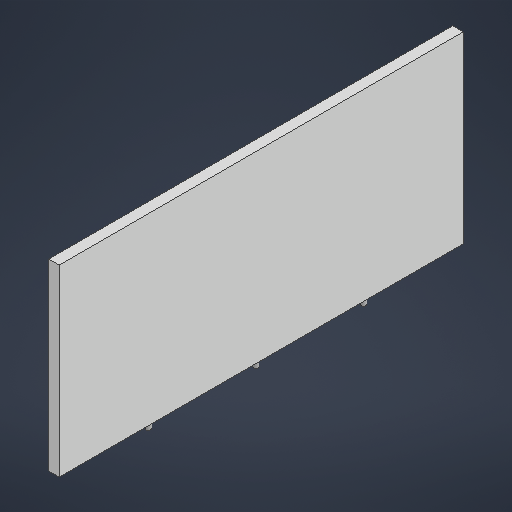
# Autodesk Inventor part: DindingKargoKananKiri
Saved by Autodesk Inventor 2026.1 (Build 301233020, 233B)
## iProperties
Created: 2025-11-09
Part Number: DindingKargoKananKiri
Material: Generic
Document SubType Name: Modeling
Designer: FrianVex
Density: 1 g/cm^3
Appearance: Default
Author: FrianVex
Autodesk Inventor part; units mm, degrees
ref_plane "YZ Plane" through (0, 0, 0) normal (1, 0, 0) x (0, 1, 0)
ref_plane "XZ Plane" through (0, 0, 0) normal (0, 1, 0) x (-1, 0, 0)
ref_plane "XY Plane" through (0, 0, 0) normal (0, 0, 1) x (1, 0, 0)
sketch "Sketch1" plane through (0, 0, 0) normal (0, 1, 0) x (-1, 0, 0)
  line L0 (2, 77) -> (-2, 77)
  line L1 (-2, 77) -> (-2, -77)
  line L2 (-2, -77) -> (2, -77)
  line L3 (2, -77) -> (2, 77)
  line L4 (2, 77) -> (-2, -77) construction
  line L5 (-2, 77) -> (2, -77) construction
  circle A0 centre (0, -41) radius 0.85
  circle A1 centre (0, 0) radius 0.85
  circle A2 centre (0, 41) radius 0.85
  point P0 (0, 0)
  dimension "d0" = 154
  dimension "d1" = 4
  dimension "d2" = 1.7
  dimension "d3" = 2
  dimension "d4" = 36
  dimension "d5" = 1.7
  dimension "d6" = 2
  dimension "d8" = 77
  dimension "d9" = 1.7
  dimension "d10" = 2
  dimension "d11" = 118
  constraints: 12 end point, 3 centre point, 2 midpoint, 2 parallel, 1 horizontal, 1 perpendicular
  measures "d0" distance of L1.end L0.end
  measures "d1" distance of L0.start L0.end
  measures "d2" diameter of A0
  measures "d3" distance from line of L3 A0.centre
  measures "d4" distance from line of L2 A0.centre
  measures "d5" diameter of A1
  measures "d6" distance from line of L3 A1.centre
  measures "d8" distance from line of L2 A1.centre
  measures "d9" diameter of A2
  measures "d10" distance from line of L3 A2.centre
  measures "d11" distance from line of L2 A2.centre
extrude "MainBody" add sketch "Sketch1" along normal blind 70
sketch "Sketch2" plane through (0, 0, 0) normal (0, -1, 0) x (1, 0, 0)
  circle A0 centre (0, 0) radius 0.85
  constraints: 1 centre point, 1 coincident
extrude "MiddlePole" add sketch "Sketch2" along normal blind 3 and the other way blind 70
sketch "Sketch3" plane through (0, 0, 0) normal (0, -1, 0) x (1, 0, 0)
  circle A0 centre (0, 41) radius 0.85 projected
  circle A1 centre (0, 41) radius 0.85
  point P0 (0, 0)
  constraints: 1 centre point, 1 coincident
extrude "UpperPole" add sketch "Sketch3" along normal blind 3 and the other way blind 70
sketch "Sketch4" plane through (0, 0, 0) normal (0, -1, 0) x (1, 0, 0)
  circle A0 centre (0, -41) radius 0.85
  point P0 (0, 0)
  constraints: 1 centre point
extrude "LowerPole" add sketch "Sketch4" along normal blind 3 and the other way blind 70
body "Solid1"
